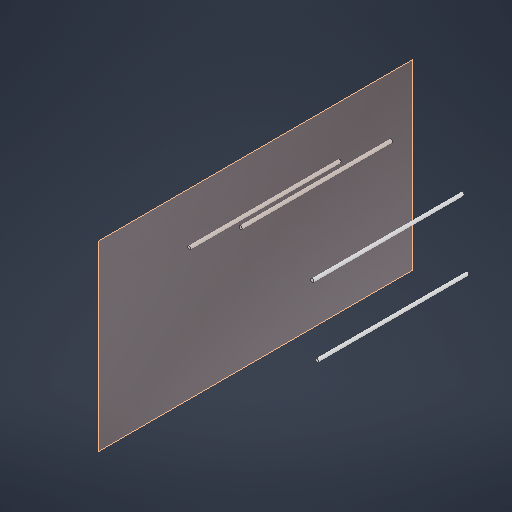
# Autodesk Inventor part: Engine_Mount_Reference_Model_V1
Saved by Autodesk Inventor 2026.1 (Build 301233000, 233)
## iProperties
Created: 2026-07-19
Part Number: Engine_Mount_Reference_Model_V1
Material: Generic
Document SubType Name: Modeling
Designer: share
Density: 1 g/cm^3
Appearance: Default
Author: share
Autodesk Inventor part; units mm, degrees
ref_plane "XZ Plane" through (0, 0, 0) normal (0, 1, 0) x (-1, 0, 0)
ref_plane "Reference Plane" through (0, 0, -100) normal (0, 0, 1) x (1, 0, 0)
sketch "Reference Image" plane through (0, 0, -100) normal (0, 0, 1) x (1, 0, 0)
  line L0 (-272, 203) -> (280.3854, 203) construction
  line L1 (280.3854, 203) -> (280.3854, -210.4856) construction
  line L2 (280.3854, -210.4856) -> (-272, -210.4856) construction
  line L3 (-272, -210.4856) -> (-272, 203) construction
  line L4 (280.3854, 203) -> (-272, -210.4856) construction
  line L5 (-382.4771, 0) -> (390.8625, 0) construction
  line L6 (0, 285.6971) -> (0, -293.1827) construction
  point P0 (0, 0)
  dimension "d26" = 690
  dimension "d51" = 203
  dimension "d54" = 272
  constraints: 2 end point, 2 other
  measures "d26" distance of L0.end L2.end
  measures "d51" distance between parallel lines of L5 L0
  measures "d54" distance between parallel lines of L6 L3
sketch "Mount Reference Sketch" plane through (0, 0, -100) normal (0, 0, 1) x (1, 0, 0)
  line L0 (-157.9294, -62) -> (-30, 45.3455) construction
  line L1 (0, 285.6971) -> (0, -293.1827) construction
  line L2 (-382.4771, 0) -> (390.8625, 0) construction
  line L3 (149, 20.5932) -> (160.6493, -146) construction
  point P0 (0, 0)
  dimension "d55" = 167
  dimension "d56" = 62
  dimension "d57" = 30
  dimension "d58" = 40
  dimension "d59" = 167
  dimension "d60" = 149
  dimension "d61" = 146
  dimension "d63" = 4
  constraints: 4 end point
  measures "d55" distance of L0.start L0.end
  measures "d56" distance from line of L2 L0.start
  measures "d57" distance from line of L0.end L1
  measures "d58" angle of L0 L2
  measures "d59" distance of L3.start L3.end
  measures "d60" distance from line of L1 L3.start
  measures "d61" distance from line of L2 L3.end
  measures "d63" angle of L3 L1
ref_plane "Mount Plane" through (0, 0, -200) normal (0, 0, 1) x (1, 0, 0)
sketch "Sketch4" plane through (0, 0, -200) normal (0, 0, 1) x (1, 0, 0)
  circle A0 centre (-30, 45.3455) radius 4
  circle A1 centre (-157.9294, -62) radius 4
  circle A2 centre (149, 20.5932) radius 4
  circle A3 centre (160.6493, -146) radius 4
  point P0 (0, 0)
  dimension "d67" = 8
  constraints: 4 centre point, 4 coincident, 3 equal radius
  measures "d67" diameter of A0
extrude "Mount XY Axes" add sketch "Sketch4" against normal blind 375
sketch "Sketch5" plane through (0, 0, -200) normal (0, 0, 1) x (1, 0, 0)
  circle A0 centre (-25, -125) radius 84
  circle A1 centre (143, -66) radius 37.5
  line L0 (-382.4771, 0) -> (390.8625, 0) projected
  line L1 (0, 285.6971) -> (0, -293.1827) projected
  line L2 (-220.7259, 38.2795) -> (-109, -125)
  line L3 (-102.1982, 130.9826) -> (21.1457, -54.8104)
  line L4 (-102.1982, 130.9826) -> (-220.7259, 38.2795)
  circle A2 centre (149, 20.5932) radius 4 projected
  line L5 (21.1457, -54.8104) -> (149, 20.5932)
  line L6 (149, 20.5932) -> (153, -132.2859)
  line L7 (153, -132.2859) -> (58.431, -134.7602)
  point P0 (0, 0)
  point P1 (152.2167, -102.3497)
  point P2 (150.3033, -29.218)
  point P3 (149.1046, 16.5946)
  point P4 (145.5546, 18.5612)
  dimension "d70" = 168
  dimension "d71" = 125
  dimension "d72" = 25
  dimension "d73" = 75
  dimension "d74" = 66
  dimension "d75" = 143
  constraints: 12 end point, 3 point on circle, 2 centre point, 1 perpendicular
  measures "d70" diameter of A0
  measures "d71" distance from line of L0 A0.centre
  measures "d72" distance from line of L1 A0.centre
  measures "d73" diameter of A1
  measures "d74" distance from line of A1.centre L0
  measures "d75" distance from line of L1 A1.centre
extrude "ROUGH Engine Block" [suppressed]
body "Solid1"
